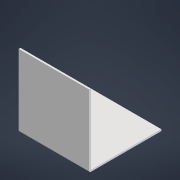
# Autodesk Inventor part: l bracket
Saved by Autodesk Inventor 2021 (Build 250183000, 183)
## iProperties
Created: 2022-05-21
Part Number: l bracket
Material: Stainless Steel
Document SubType Name: Modeling
Designer: techv
Mass: 3.23142 g
Surface Area: 16.761 cm^2
Volume: 0.403927 cm^3
Density: 8 g/cm^3
Appearance: Semi-Polished
Author: techv
Autodesk Inventor part; units mm, degrees
ref_plane "YZ Plane" through (0, 0, 0) normal (1, 0, 0) x (0, 1, 0)
ref_plane "XZ Plane" through (0, 0, 0) normal (0, 1, 0) x (-1, 0, 0)
ref_plane "XY Plane" through (0, 0, 0) normal (0, 0, 1) x (1, 0, 0)
sketch "Sketch1" plane through (0, 0, 0) normal (0, 1, 0) x (-1, 0, 0)
  line L0 (-10, 10) -> (10, 10)
  line L1 (10, 10) -> (10, -10)
  line L2 (10, -10) -> (-10, -10)
  line L3 (-10, -10) -> (-10, 10)
  line L4 (-10, 10) -> (10, -10) construction
  line L5 (10, 10) -> (-10, -10) construction
  point P0 (0, 0)
  dimension "d0" = 20
  dimension "d1" = 20
  constraints: 12 end point, 2 midpoint, 2 parallel, 1 horizontal, 1 perpendicular
  measures "d0" distance of L1.end L2.end
  measures "d1" distance of L0.end L1.end
extrude "Extrusion1" add sketch "Sketch1" along normal blind 0.5
sketch "Sketch2" plane through (0, 0.5, 0) normal (0, 1, 0) x (1, 0, 0)
  line L0 (10, 10) -> (-10, 10) projected
  line L1 (-10, 10) -> (-10, -10) projected
  line L2 (-10, -10) -> (10, -10) projected
  line L3 (10, -10) -> (10, 10) projected
  line L4 (-10, -10) -> (10, -10) projected
  line L5 (10, -10) -> (-10, -10)
  line L6 (-10, -10) -> (-10, -10.5)
  line L7 (-10, -10.5) -> (10, -10.5)
  line L8 (10, -10.5) -> (10, -10)
  point P0 (0, 0)
  dimension "d4" = 0.5
  constraints: 8 end point, 2 parallel, 1 horizontal, 1 perpendicular
  measures "d4" distance of L6.end L5.end
extrude "Extrusion2" add sketch "Sketch2" along normal blind 20 contours L8 L7 L6 L2
sketch "Sketch3" plane through (10, 0.5, 10.5) normal (1, 0, 0) x (0, 0, -1)
  line L0 (0.5, 0) -> (20.5, 0) projected
  line L1 (0.5, -0.5) -> (0.5, 0) projected
  circle A0 centre (0.5, 0) radius 0.5
  line L2 (0, 0) -> (0.5, 0) projected
  line L3 (0.5, 0) -> (0.5, 20) projected
  line L4 (0, 20) -> (0.5, 20) projected
  line L5 (0, 0) -> (0, 20) projected
  point P0 (10.5, -0.5)
  constraints: 3 other
extrude "Extrusion3" add sketch "Sketch3" against normal up to surface (20 mm away) contours L1 A0 L2
sketch "Sketch4" plane through (0, 0.5, 0) normal (0, 1, 0) x (1, 0, 0)
  point P0 (0, 0)
body "Solid1"
